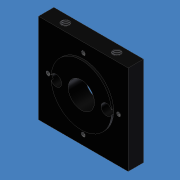
# Autodesk Inventor part: BB1-BackPlate
Saved by Autodesk Inventor 2015 (Build 190159000, 159)
## iProperties
Company: FirstCadLibrary
Shininess: 64.0
Length Units: 11269
Angle Units: 11279
Time Units: 11290
Mass Units: 11283
Length Display Precision: 3
Angle Display Precision: 2
Compacted: True
Part Number: BB1-BackPlate
Document SubType Name: Modeling
Created: 2007-01-08
Material: Steel, Mild
Designer: Ed Sparks
Catalog Web Link: www.banebots.com
Vendor: BaneBots
Density: 1 g/cm^3
Appearance: Anodized - Black
Density: 0.0
Volumn: 0.0
Area: 0.0
PropertySet Name: Model Information
Control State: 0
Master: False
Checked Out: False
Author: Ed Sparks
Autodesk Inventor part; units mm, degrees
ref_plane "YZ Plane" through (0, 0, 0) normal (1, 0, 0) x (0, 1, 0)
ref_plane "XZ Plane" through (0, 0, 0) normal (0, 1, 0) x (-1, 0, 0)
ref_plane "XY Plane" through (0, 0, 0) normal (0, 0, 1) x (1, 0, 0)
sketch "Sketch1" plane through (0, 0, 0) normal (0, 0, 1) x (1, 0, 0)
  line L0 (-22.225, 22.225) -> (22.225, 22.225)
  line L1 (22.225, 22.225) -> (22.225, -22.225)
  line L2 (22.225, -22.225) -> (-22.225, -22.225)
  line L3 (-22.225, -22.225) -> (-22.225, 22.225)
  line L4 (0, 0) -> (0, 22.225) construction
  line L5 (0, 0) -> (0, -22.225) construction
  line L6 (0, 0) -> (22.225, 0) construction
  line L7 (0, 0) -> (-22.225, 0) construction
  dimension "d0" = 44.45
  dimension "d1" = 44.45
  constraints: 16 end point, 4 midpoint, 3 perpendicular, 2 collinear, 2 parallel, 1 horizontal, 1 other
  measures "d0" distance of L0.start L0.end
  measures "d1" distance of L0.end L1.end
extrude "Extrusion1" add sketch "Sketch1" along normal mid plane 7.62
sketch "Sketch2" plane through (0, 0, -3.81) normal (0, 0, -1) x (-1, 0, 0)
  point P0 (0, 0)
  constraints: 1 other
hole "Hole1" at (0, 0, -3.81) direction (0, 0, 1) diameter 13 end through all
sketch "Sketch7" plane through (0, 0, -3.81) normal (0, 0, -1) x (-1, 0, 0)
  circle A0 centre (0, 0) radius 6.5 projected
  circle A1 centre (0, 0) radius 15
  dimension "d49" = 30
  constraints: 1 centre point, 1 coincident, 1 concentric
  measures "d49" diameter of A1
extrude "Extrusion2" add sketch "Sketch7" along normal blind 1
sketch "Sketch8" plane through (0, 0, 3.81) normal (0, 0, 1) x (1, 0, 0)
  circle A0 centre (0, 0) radius 6.5 projected
  line L0 (22.225, -22.225) -> (-22.225, -22.225) projected
  line L1 (0, 0) -> (26.1346, 0) construction
  line L2 (0, 0) -> (0, -12.5) construction
  dimension "d52" = 90
  dimension "d53" = 12.5
  constraints: 4 end point, 1 parallel
  measures "d52" angle of L1 L2
  measures "d53" distance of L1.start L2.end
hole "Hole6" at (0, -12.5, 3.81) direction (0, 0, -1) diameter 3 end through all
sketch "Sketch9" plane through (0, 0, -4.81) normal (0, 0, -1) x (-1, 0, 0)
  arc A0 (-7.7164, -9.8339) -> (-9.8339, -7.7164) centre (0, -12.5) ccw projected
  point P0 (0, -12.5)
  constraints: 1 coincident, 1 other
hole "Hole7" at (0, -12.5, -4.81) direction (0, 0, 1) diameter 5.4 depth 5.5 tip angle 118
pattern_circular "Circular Pattern2" count 2 over 360 about axis through (0, 0, 59.512) along (0, 0, -1) of "Hole6", "Hole7"
sketch "Sketch10" plane through (0, 0, -3.81) normal (0, 0, -1) x (-1, 0, 0)
  arc A0 (1.1164, -14.9584) -> (1.1164, 14.9584) centre (0, 0) ccw projected
  point P0 (0, 17.5)
  dimension "d71" = 17.5
  constraints: 1 vertical alignment
  measures "d71" distance of point (0, 17.5) A0.centre
hole "Hole8" at (0, 17.5, -3.81) direction (0, 0, 1) diameter 2.013 end through all thread size "M2.5x0.45" class "6H" standard "ANSI Metric M Profile"
pattern_circular "Circular Pattern3" count 4 over 360 about axis through (0, 0, 59.512) along (0, 0, -1) of "Hole8"
sketch "Sketch11" plane through (22.225, -22.225, 3.81) normal (1, 0, 0) x (0, 0, -1)
  line L0 (0, 44.45) -> (0, 0) projected
  line L1 (0, 0) -> (7.62, 0) projected
  line L2 (7.62, 0) -> (7.62, 44.45) projected
  line L3 (0, 44.45) -> (7.62, 44.45) projected
  line L4 (3.81, 0) -> (3.81, 44.45) construction
  line L5 (7.62, 22.225) -> (0, 22.225) construction
  point P0 (3.81, 9.525)
  dimension "d82" = 12.7
  constraints: 4 end point, 4 midpoint, 1 point on line
  measures "d82" distance from line of L5 point (3.81, 9.525)
hole "Hole9" at (22.225, -12.7, 0) direction (-1, 0, 0) diameter 3.962 depth 10 tip angle 118 thread size "10-32 UNF" class "2B" standard "ANSI Unified Screw Threads"
mirror "Mirror7" about plane through (0, 0, 0) normal (0, 1, 0) of "Hole9"
mirror "Mirror8" about plane through (0, 0, 0) normal (1, 0, 0) of "Hole9", "Mirror7"
body "Solid1"
